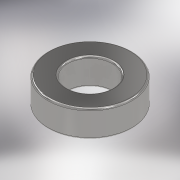
# Autodesk Inventor part: ThrustBearing_OD_47_ID_25_W_15
Saved by Autodesk Inventor 2020.3 (Build 243373000, 373)
## iProperties
Created: 2021-08-03
Part Number: ThrustBearing_OD_47_ID_25_W_15
Material: Steel
Document SubType Name: Modeling
Designer: justi
Density: 7.85 g/cm^3
Appearance: Steel - Polished
Author: justi
Autodesk Inventor part; units mm, degrees
ref_plane "YZ Plane" through (0, 0, 0) normal (1, 0, 0) x (0, 1, 0)
ref_plane "XZ Plane" through (0, 0, 0) normal (0, 1, 0) x (-1, 0, 0)
ref_plane "XY Plane" through (0, 0, 0) normal (0, 0, 1) x (1, 0, 0)
sketch "Sketch1" plane through (0, 0, 0) normal (0, 1, 0) x (-1, 0, 0)
  circle A0 centre (0, 0) radius 12.5
  circle A1 centre (0, 0) radius 23.5
  dimension "d0" = 25
  dimension "d1" = 47
  constraints: 2 centre point, 2 coincident
  measures "d0" diameter of A0
  measures "d1" diameter of A1
extrude "Extrusion1" add sketch "Sketch1" along normal blind 15
fillet "Fillet1" radius 1 4 edges at (12.5, 15, 0) (12.5, 0, 0) (23.5, 0, 0) (23.5, 15, 0)
body "Solid1"
